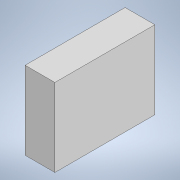
# Autodesk Inventor part: block_1
Saved by Autodesk Inventor 2020.1 (Build 241239000, 239)
## iProperties
Created: 2020-01-22
Part Number: block_1
Material: Generic
Document SubType Name: Modeling
Designer: Ali
Density: 1 g/cm^3
Appearance: Default
Author: Ali
Autodesk Inventor part; units mm, degrees
ref_plane "YZ Plane" through (0, 0, 0) normal (1, 0, 0) x (0, 1, 0)
ref_plane "XZ Plane" through (0, 0, 0) normal (0, 1, 0) x (-1, 0, 0)
ref_plane "XY Plane" through (0, 0, 0) normal (0, 0, 1) x (1, 0, 0)
sketch "Sketch1" plane through (0, 0, 0) normal (0, 0, 1) x (1, 0, 0)
  line L0 (0, 0) -> (1.49, 0)
  line L1 (1.49, 0) -> (1.49, -3.9)
  line L2 (1.49, -3.9) -> (0, -3.9)
  line L3 (0, -3.9) -> (0, 0)
  dimension "d0" = 1.49
  dimension "d1" = 3.9
  constraints: 8 end point, 2 parallel, 1 horizontal, 1 perpendicular
  measures "d0" distance of L0.start L0.end
  measures "d1" distance of L2.end L0.start
extrude "Extrusion1" add sketch "Sketch1" along normal blind 5
equation "\"d2\" = OG_shaftLength"
equation "\"Wheel_Related_W_\" = 0"
equation "\"W_innerDiameter\" = 35"
equation "\"W_innerDepth\" = 4.5"
equation "\"W_wallThickness\" = 1"
equation "\"W_holesClearance\" = 0.3"
equation "\"W_outerGearHoleDiameter\" = 2.1"
equation "\"W_innerGearHoleDiameter\" = 5.1"
equation "\"TempSpotReserved7\" = 0"
equation "\"TempSpotReserved8\" = 0"
equation "\"TempSpotReserved9\" = 0"
equation "\"TempSpotReserved10\" = 0"
equation "\"Inner_Gear_Related_IG_\" = 0"
equation "\"IG_shaftDiameter\" = 2.5"
equation "\"IG_gearThickness\" = 1"
equation "\"IG_skirtOffset\" = 1.5"
equation "\"IG_skirtThickness\" = 0.5"
equation "\"IG_extentionLength\" = 7"
equation "\"IG_extentionThickness\" = 1"
equation "\"IG_slitWidth\" = 1.5"
equation "\"IG_slitlength\" = 4"
equation "\"Outer_Gear_Related_OG_\" = 0"
equation "\"OG_shaftDiameter\" = 1.5"
equation "\"OG_shaftLength\" = 5"
equation "\"OG_gearThickness\" = 1"
equation "\"OG_skirtOffset\" = 1"
equation "\"OG_skirtThickness\" = 1"
equation "\"TempSpotReserved29\" = 0"
equation "\"TempSpotReserved30\" = 0"
equation "\"Leg_Extensions_Related_LE_\" = 0"
equation "\"LE_baseDiameter\" = 2"
equation "\"LE_maxLength\" = 10.64459"
equation "\"LE_thickness\" = 2"
equation "\"LE_offsetAboveOuterGear\" = 0"
equation "\"TempSpotReserved35\" = 0"
equation "\"TempSpotReserved36\" = 0"
equation "\"TempSpotReserved37\" = 0"
equation "\"TempSpotReserved38\" = 0"
equation "\"TempSpotReserved39\" = 0"
equation "\"TempSpotReserved40\" = 0"
equation "\"Bearing_Related_B_\" = 0"
equation "\"B_bearingThickness\" = 1"
equation "\"TempSpotReserved42\" = 0"
equation "\"TempSpotReserved43\" = 0"
equation "\"TempSpotReserved44\" = 0"
equation "\"TempSpotReserved45\" = 0"
equation "\"TempSpotReserved46\" = 0"
equation "\"TempSpotReserved47\" = 0"
equation "\"TempSpotReserved48\" = 0"
equation "\"TempSpotReserved49\" = 0"
equation "\"TempSpotReserved50\" = 0"
body "Solid1"
